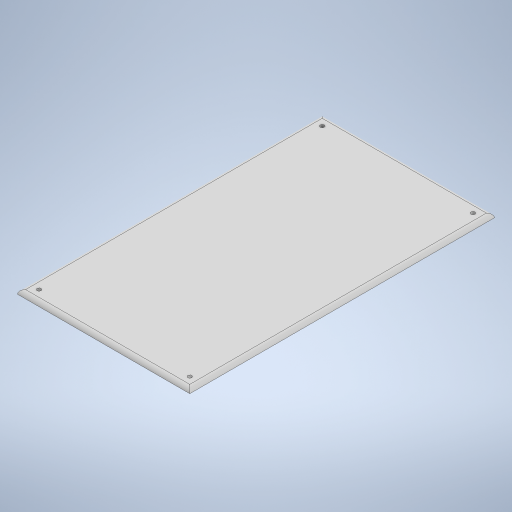
# Autodesk Inventor part: Lid
Saved by Autodesk Inventor 2023 (Build 270158000, 158)
## iProperties
Created: 2023-01-17
Part Number: Lid
Material: Generic
Document SubType Name: Modeling
Designer: Ahmed Nazir
Density: 1 g/cm^3
Appearance: Default
Author: Ahmed Nazir
Autodesk Inventor part; units mm, degrees
ref_plane "YZ Plane" through (0, 0, 0) normal (1, 0, 0) x (0, 1, 0)
ref_plane "XZ Plane" through (0, 0, 0) normal (0, 1, 0) x (-1, 0, 0)
ref_plane "XY Plane" through (0, 0, 0) normal (0, 0, 1) x (1, 0, 0)
sketch "Sketch1" plane through (0, 0, 0) normal (0, 1, 0) x (-1, 0, 0)
  line L0 (0, 0) -> (-127.76, 0)
  line L1 (-127.76, 0) -> (-127.76, -226)
  line L2 (-127.76, -226) -> (0, -226)
  line L3 (0, -226) -> (0, 0)
  line L4 (-3, -3) -> (-124.76, -3)
  line L5 (-124.76, -3) -> (-124.76, -223)
  line L6 (-124.76, -223) -> (-3, -223)
  line L7 (-3, -223) -> (-3, -3)
  dimension "d0" = 127.76
  dimension "d1" = 226
  dimension "d2" = 3
  constraints: 16 end point, 4 parallel, 2 perpendicular, 1 horizontal, 3 other
  measures "d0" distance of L2.end L1.end
  measures "d1" distance of L1.end L0.end
  measures "d2" distance between parallel lines of L3 L7
extrude "Extrusion1" add sketch "Sketch1" against normal blind 3 contours L7 L6 L5 L4
extrude "Extrusion2" add sketch "Sketch1" along normal blind 3 contours L3 L2 L1 L0 | L7 L6 L5 L4
sketch "Sketch2" plane through (0, 3, 0) normal (0, 1, 0) x (1, 0, 0)
  line L0 (0, 226) -> (0, 0) projected
  line L1 (0, 113) -> (127.76, 113) construction
  line L2 (127.76, 0) -> (127.76, 226) projected
  line L3 (0, 0) -> (127.76, 0) projected
  line L4 (63.88, 0) -> (63.88, 226) construction
  line L5 (127.76, 226) -> (0, 226) projected
  circle A0 centre (119.76, 8) radius 1.5
  circle A1 centre (8, 8) radius 1.5
  circle A2 centre (119.76, 218) radius 1.5
  circle A3 centre (8, 218) radius 1.5
  dimension "d7" = 3
  dimension "d8" = 8
  dimension "d9" = 8
  constraints: 4 centre point, 4 end point, 4 midpoint, 3 symmetric about line, 3 other
  measures "d7" diameter of A0
  measures "d8" distance from line of L2 A0.centre
  measures "d9" distance from line of L3 A0.centre
extrude "Extrusion3" cut sketch "Sketch2" against normal through all contours A0 | A1 | A2 | A3
fillet "Fillet1" radius 3 4 edges at (127.76, 3, -113) (63.88, 3, -226) (0, 3, -113) (63.88, 3, 0)
body "Solid1"
